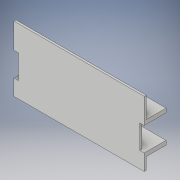
# Autodesk Inventor part: Part1
Saved by Autodesk Inventor 2019 (Build 230136000, 136)
## iProperties
Created: 2019-12-09
Part Number: Part1
Material: Generic
Document SubType Name: Modeling
Designer: ABHISHEK
Density: 1 g/cm^3
Appearance: Default
Author: ABHISHEK
Autodesk Inventor part; units mm, degrees
ref_plane "YZ Plane" through (0, 0, 0) normal (1, 0, 0) x (0, 1, 0)
ref_plane "XZ Plane" through (0, 0, 0) normal (0, 1, 0) x (-1, 0, 0)
ref_plane "XY Plane" through (0, 0, 0) normal (0, 0, 1) x (1, 0, 0)
sketch "Sketch1" plane through (0, 0, 0) normal (0, 0, 1) x (1, 0, 0)
  line L0 (-17.8746, 7.514) -> (482.1254, 7.514)
  line L1 (482.1254, 7.514) -> (482.1254, -242.486)
  line L2 (482.1254, -242.486) -> (-17.8746, -242.486)
  line L3 (-17.8746, -242.486) -> (-17.8746, 7.514)
  point P0 (0, 0)
  dimension "d0" = 500
  dimension "d1" = 250
  constraints: 8 end point, 2 parallel, 1 horizontal, 1 perpendicular
  measures "d0" distance of L1.end L2.end
  measures "d1" distance of L0.end L1.end
extrude "Extrusion1" add sketch "Sketch1" along normal blind 8
sketch "Sketch2" plane through (0, 0, 0) normal (0, 0, -1) x (-1, 0, 0)
  point P0 (0, 0)
sketch "Sketch3" plane through (0, 0, 0) normal (0, 0, -1) x (-1, 0, 0)
  line L0 (17.8746, 7.514) -> (17.8746, -242.486) projected
  line L1 (0, -89.2163) -> (17.8746, -89.2163)
  line L2 (17.8746, -89.2163) -> (17.8746, -180.8626)
  line L3 (17.8746, -180.8626) -> (0, -180.8626)
  line L4 (0, -180.8626) -> (0, -89.2163)
  line L5 (-482.1254, -242.486) -> (-482.1254, 7.514) projected
  line L6 (-465.1744, -89.2163) -> (-482.1254, -89.2163)
  line L7 (-482.1254, -89.2163) -> (-482.1254, -180.8626)
  line L8 (-482.1254, -180.8626) -> (-465.1744, -180.8626)
  line L9 (-465.1744, -180.8626) -> (-465.1744, -89.2163)
  point P0 (0, 0)
  constraints: 16 end point, 4 parallel, 4 point on line, 2 horizontal, 2 perpendicular
extrude "Extrusion2" cut sketch "Sketch3" against normal blind 8
sketch "Sketch4" plane through (0, 0, 0) normal (0, 0, -1) x (-1, 0, 0)
  line L0 (17.8746, -89.2163) -> (17.8746, 7.514) projected
  line L1 (17.8746, -73.5948) -> (-191.2332, -73.5948)
  line L2 (-191.2332, -73.5948) -> (-191.2332, -89.2163)
  line L3 (-191.2332, -89.2163) -> (17.8746, -89.2163)
  line L4 (17.8746, -89.2163) -> (17.8746, -73.5948)
  line L5 (17.8746, -180.8626) -> (0, -180.8626) projected
  line L6 (17.8746, -180.8626) -> (-191.2332, -180.8626)
  line L7 (-191.2332, -180.8626) -> (-191.2332, -196.8404)
  line L8 (-191.2332, -196.8404) -> (17.8746, -196.8404)
  line L9 (17.8746, -196.8404) -> (17.8746, -180.8626)
  line L10 (-482.1254, 7.514) -> (-482.1254, -89.2163) projected
  line L11 (-482.1254, -89.2163) -> (-286.3362, -89.2163)
  line L12 (-286.3362, -89.2163) -> (-286.3362, -73.5948)
  line L13 (-286.3362, -73.5948) -> (-482.1254, -73.5948)
  line L14 (-482.1254, -73.5948) -> (-482.1254, -89.2163)
  line L15 (-482.1254, -180.8626) -> (-482.1254, -242.486) projected
  line L16 (-286.3362, -180.8626) -> (-482.1254, -180.8626)
  line L17 (-482.1254, -180.8626) -> (-482.1254, -196.8404)
  line L18 (-482.1254, -196.8404) -> (-286.3362, -196.8404)
  line L19 (-286.3362, -196.8404) -> (-286.3362, -180.8626)
  point P0 (0, 0)
  constraints: 32 end point, 8 parallel, 7 point on line, 4 horizontal, 4 perpendicular
extrude "Extrusion3" add sketch "Sketch4" along normal blind 76.2
body "Solid1"
